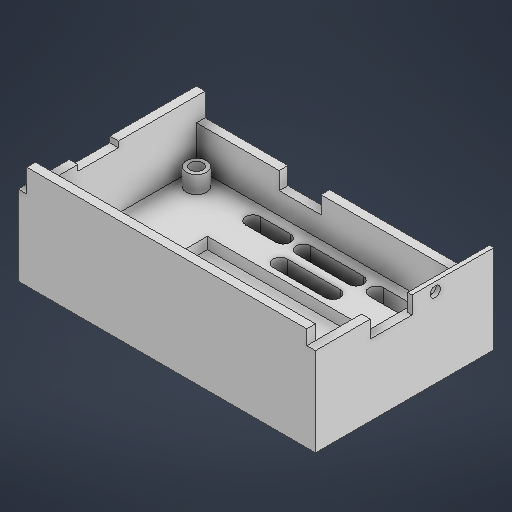
# Autodesk Inventor part: krabice
Saved by Autodesk Inventor 2025 (Build 290162000, 162)
## iProperties
Created: 2025-01-29
Part Number: krabice
Material: Všeobecné
Document SubType Name: Modeling
Designer: psutk
Density: 1 g/cm^3
Appearance: Výchozí
Author: psutk
Autodesk Inventor part; units mm, degrees
ref_plane "YZ Plane" through (0, 0, 0) normal (1, 0, 0) x (0, 1, 0)
ref_plane "XZ Plane" through (0, 0, 0) normal (0, 1, 0) x (-1, 0, 0)
ref_plane "XY Plane" through (0, 0, 0) normal (0, 0, 1) x (1, 0, 0)
sketch "Náčrt1" plane through (0, 0, 0) normal (0, 0, 1) x (1, 0, 0)
  line L0 (-47.25, 26.75) -> (47.25, 26.75)
  line L1 (47.25, 26.75) -> (47.25, -26.75)
  line L2 (47.25, -26.75) -> (-47.25, -26.75)
  line L3 (-47.25, -26.75) -> (-47.25, 26.75)
  line L4 (0, 43.05) -> (0, -43.05) projected
  line L5 (-71.75, 0) -> (71.75, 0) projected
  line L6 (51.25, 30.75) -> (-51.25, 30.75)
  line L7 (-51.25, 30.75) -> (-51.25, -30.75)
  line L8 (-51.25, -30.75) -> (51.25, -30.75)
  line L9 (51.25, -30.75) -> (51.25, 30.75)
  point P0 (0, 0)
  dimension "d0" = 94.5
  dimension "d1" = 53.5
  dimension "d2" = 4
  constraints: 16 end point, 4 parallel, 2 perpendicular, 1 horizontal, 5 other
  measures "d0" distance of L1.end L2.end
  measures "d1" distance of L0.end L1.end
  measures "d2" distance between parallel lines of L0 L6
extrude "Vysunutí1" add sketch "Náčrt1" along normal blind 4
sketch "Náčrt5" plane through (0, 0, 0) normal (0, 0, -1) x (-1, 0, 0)
  line L0 (51.25, -30.75) -> (-51.25, -30.75) projected
  line L1 (-51.25, -30.75) -> (-51.25, 30.75) projected
  line L2 (51.25, -30.75) -> (-51.25, -30.75)
  line L3 (-51.25, -30.75) -> (-51.25, 30.75)
  line L4 (-51.25, 30.75) -> (51.25, 30.75)
  line L5 (51.25, 30.75) -> (51.25, -30.75)
  line L6 (51.25, -30.75) -> (-51.25, -30.75) projected
  line L7 (51.25, 30.75) -> (51.25, -30.75) projected
  line L8 (-51.25, 30.75) -> (51.25, 30.75) projected
  line L9 (-51.25, -30.75) -> (-51.25, 30.75) projected
  point P0 (0, 0)
  point P1 (42.75, -22.25)
  constraints: 8 end point, 2 parallel, 1 horizontal, 1 perpendicular
extrude "Vysunutí4" add sketch "Náčrt5" along normal blind 2
sketch "Náčrt7" plane through (0, 0, 4) normal (0, 0, 1) x (1, 0, 0)
  line L0 (-51.25, -30.75) -> (51.25, -30.75) projected
  line L1 (51.25, -30.75) -> (51.25, 30.75) projected
  line L2 (51.25, 30.75) -> (-51.25, 30.75) projected
  line L3 (-51.25, 30.75) -> (-51.25, -30.75) projected
  line L4 (-48.25, 27.75) -> (48.25, 27.75)
  line L5 (48.25, 27.75) -> (48.25, -27.75)
  line L6 (48.25, -27.75) -> (-48.25, -27.75)
  line L7 (-48.25, -27.75) -> (-48.25, 27.75)
  point P0 (0, 0)
  dimension "d44" = 61.5
  dimension "d45" = 102.5
  dimension "d46" = 3
  dimension "d47" = 3
  dimension "d48" = 3
  dimension "d49" = 3
  constraints: 8 end point, 2 parallel, 1 horizontal, 1 perpendicular
  measures "d44" distance of L2.end L0.start
  measures "d45" distance of L1.end L2.end
  measures "d46" distance between parallel lines of L2 L4
  measures "d47" distance between parallel lines of L3 L7
  measures "d48" distance between parallel lines of L1 L5
  measures "d49" distance between parallel lines of L0 L6
extrude "Vysunutí5" add sketch "Náčrt7" along normal blind 7.5
sketch "Náčrt8" plane through (0, 0, 11.5) normal (0, 0, 1) x (1, 0, 0)
  line L0 (48.25, -27.75) -> (48.25, 27.75) projected
  line L1 (-51.25, 30.75) -> (51.25, 30.75) projected
  line L2 (48.25, 27.75) -> (-5.34, 27.75)
  line L3 (-5.34, 27.75) -> (-5.34, 30.75)
  line L4 (-5.34, 30.75) -> (48.25, 30.75)
  line L5 (48.25, 30.75) -> (48.25, 27.75)
  line L6 (48.25, 27.75) -> (-48.25, 27.75) projected
  line L7 (-48.25, 27.75) -> (-19.76, 27.75)
  line L8 (-19.76, 27.75) -> (-19.76, 30.75)
  line L9 (-19.76, 30.75) -> (-48.25, 30.75)
  line L10 (-48.25, 30.75) -> (-48.25, 27.75)
  point P0 (0, 0)
  dimension "d52" = 53.59
  dimension "d53" = 28.49
  constraints: 16 end point, 4 parallel, 2 horizontal, 2 perpendicular, 2 point on line
  measures "d52" distance of L3.end L4.end
  measures "d53" distance of L9.end L8.end
extrude "Vysunutí6" add sketch "Náčrt8" along normal blind 6 contours L1 L8 L6 L10 | L1 L5 L2 L3
sketch "Náčrt9" plane through (0, 0, 11.5) normal (0, 0, 1) x (1, 0, 0)
  line L0 (51.25, -30.75) -> (51.25, 30.75) projected
  line L1 (51.25, 30.75) -> (48.25, 30.75) projected
  line L2 (51.25, -30.75) -> (48.25, -30.75)
  line L3 (48.25, -30.75) -> (48.25, 30.75)
  line L4 (48.25, 30.75) -> (51.25, 30.75)
  line L5 (51.25, 30.75) -> (51.25, -30.75)
  point P0 (0, 0)
  constraints: 8 end point, 2 parallel, 1 horizontal, 1 perpendicular
extrude "Vysunutí7" add sketch "Náčrt9" along normal blind 11
sketch "Náčrt10" plane through (0, 0, 22.5) normal (0, 0, 1) x (1, 0, 0)
  line L0 (48.25, 30.75) -> (48.25, -30.75) projected
  line L1 (51.25, -30.75) -> (51.25, 30.75) projected
  line L2 (48.25, -11.888) -> (51.25, -11.888)
  line L3 (51.25, -11.888) -> (51.25, 2.532)
  line L4 (51.25, 2.532) -> (48.25, 2.532)
  line L5 (48.25, 2.532) -> (48.25, -11.888)
  line L6 (48.25, -4.678) -> (51.25, -4.678)
  line L7 (48.25, -30.75) -> (51.25, -30.75)
  line L8 (51.25, -30.75) -> (51.25, -11.888)
  line L9 (51.25, -11.888) -> (48.25, -11.888)
  line L10 (48.25, -11.888) -> (48.25, -30.75)
  line L11 (48.25, 2.532) -> (51.25, 2.532)
  line L12 (51.25, 2.532) -> (51.25, 30.75)
  line L13 (51.25, 30.75) -> (48.25, 30.75)
  line L14 (48.25, 30.75) -> (48.25, 2.532)
  point P0 (0, 0)
  dimension "d58" = 26.072
  dimension "d59" = 14.42
  constraints: 26 end point, 6 parallel, 4 perpendicular, 3 horizontal, 3 point on line, 1 midpoint, 1 other
  measures "d58" distance of L0.end L6.start
  measures "d59" distance of L3.end L2.end
extrude "Vysunutí8" add sketch "Náčrt10" along normal blind 6 contours L13 L1 L4 L0 | L2 L1 L7 L0
sketch "Náčrt11" plane through (0, 0, 11.5) normal (0, 0, 1) x (1, 0, 0)
  line L0 (-51.25, -30.75) -> (48.25, -30.75) projected
  line L1 (-48.25, 30.75) -> (-48.25, 27.75) projected
  line L2 (-51.25, -30.75) -> (-48.25, -30.75)
  line L3 (-48.25, -30.75) -> (-48.25, 30.75)
  line L4 (-48.25, 30.75) -> (-51.25, 30.75)
  line L5 (-51.25, 30.75) -> (-51.25, -30.75)
  point P0 (0, 0)
  constraints: 8 end point, 2 parallel, 1 horizontal, 1 perpendicular
extrude "Vysunutí9" add sketch "Náčrt11" along normal blind 12
sketch "Náčrt12" plane through (0, 0, 23.5) normal (0, 0, 1) x (1, 0, 0)
  line L0 (-51.25, -30.75) -> (-48.25, -30.75) projected
  line L1 (-48.25, -30.75) -> (-48.25, 30.75) projected
  line L2 (-48.25, 30.75) -> (-51.25, 30.75) projected
  line L3 (-51.25, 30.75) -> (-51.25, -30.75) projected
  line L4 (-48.25, -6.14) -> (-51.25, -6.14)
  line L5 (-48.25, 0.86) -> (-51.25, 0.86)
  line L6 (-51.25, 0.86) -> (-51.25, -13.14)
  line L7 (-51.25, -13.14) -> (-48.25, -13.14)
  line L8 (-48.25, -13.14) -> (-48.25, 0.86)
  line L9 (-48.25, 30.75) -> (-51.25, 30.75)
  line L10 (-51.25, 30.75) -> (-51.25, 0.86)
  line L11 (-51.25, 0.86) -> (-48.25, 0.86)
  line L12 (-48.25, 0.86) -> (-48.25, 30.75)
  line L13 (-48.25, -13.14) -> (-51.25, -13.14)
  line L14 (-51.25, -13.14) -> (-51.25, -30.75)
  line L15 (-51.25, -30.75) -> (-48.25, -30.75)
  line L16 (-48.25, -30.75) -> (-48.25, -13.14)
  point P0 (0, 0)
  point P1 (-48.25, -13.14)
  point P2 (-51.25, 0.86)
  dimension "d64" = 24.61
  dimension "d65" = 14
  constraints: 26 end point, 6 parallel, 4 perpendicular, 4 point on line, 3 horizontal, 1 other
  measures "d64" distance from line of L0 L4.start
  measures "d65" distance of L6.end L5.end
extrude "Vysunutí10" add sketch "Náčrt12" along normal blind 2 contours L3 L7 L1 L0 | L3 L2 L1 L5
sketch "Náčrt13" plane through (0, 0, 11.5) normal (0, 0, 1) x (1, 0, 0)
  line L0 (-48.25, -30.75) -> (48.25, -30.75) projected
  line L1 (-48.25, -30.75) -> (48.25, -30.75)
  line L2 (48.25, -30.75) -> (48.25, -27.75)
  line L3 (48.25, -27.75) -> (-48.25, -27.75)
  line L4 (-48.25, -27.75) -> (-48.25, -30.75)
  point P0 (0, 0)
  constraints: 8 end point, 2 parallel, 1 horizontal, 1 perpendicular
extrude "Vysunutí11" add sketch "Náčrt13" along normal blind 17
sketch "Náčrt14" plane through (0, 0, 4) normal (0, 0, 1) x (1, 0, 0)
  line L0 (-48.25, 27.75) -> (-48.25, -27.75) projected
  line L1 (-48.25, -27.75) -> (48.25, -27.75) projected
  line L2 (48.25, -27.75) -> (48.25, 27.75) projected
  line L3 (48.25, 27.75) -> (-48.25, 27.75) projected
  line L4 (0, 43.05) -> (0, -43.05) projected
  line L5 (-71.75, 0) -> (71.75, 0) projected
  line L6 (39.75, -20.5179) -> (42.75, -18.7859)
  line L7 (42.75, -18.7859) -> (45.75, -20.5179)
  line L8 (45.75, -20.5179) -> (45.75, -23.9821)
  line L9 (45.75, -23.9821) -> (42.75, -25.7141)
  line L10 (42.75, -25.7141) -> (39.75, -23.9821)
  line L11 (39.75, -23.9821) -> (39.75, -20.5179)
  point P0 (0, 0)
  point P1 (42.75, -22.25)
  point P2 (-42.75, -22.25)
  point P3 (-42.75, 22.25)
  point P4 (42.75, 22.25)
  point P5 (42.75, -22.25)
  dimension "d70" = 5.5
  dimension "d71" = 5.5
  dimension "d72" = 6
  constraints: 12 end point, 3 symmetric about line, 1 coincident, 13 other
  measures "d70" distance from line of L1 point (42.75, -22.25)
  measures "d71" distance from line of L2 point (42.75, -22.25)
  measures "d72" distance between parallel lines of L8 L11
extrude "Vysunutí12" cut sketch "Náčrt14" along normal blind 4 from surface at -6 contours L6 L7 L8 L9 L10 L11
pattern_linear "Obdélníkové pole3" count 2 spacing 85.5 along (-1, 0, 0) count 2 spacing 44.5 along (0, 1, 0) of "Vysunutí12"
sketch "Náčrt16" plane through (0, 0, 4) normal (0, 0, 1) x (1, 0, 0)
  circle A0 centre (42.75, -22.25) radius 1.7 projected
  circle A1 centre (42.75, -22.25) radius 3.5
  point P0 (0, 0)
  dimension "d115" = 7
  constraints: 2 coincident, 1 centre point
  measures "d115" diameter of A1
extrude "Vysunutí13" add sketch "Náčrt16" along normal blind 6 contours A0 | A1
pattern_linear "Obdélníkové pole5" count 2 spacing 85.5 along (-1, 0, 0) count 2 spacing 44.5 along (0, 1, 0) of "Vysunutí13"
sketch "Náčrt17" plane through (0, 0, 10) normal (0, 0, 1) x (1, 0, 0)
  line L0 (39.5, -24.1264) -> (42.75, -26.0028) projected
  line L1 (42.75, -26.0028) -> (46, -24.1264) projected
  line L2 (46, -24.1264) -> (46, -20.3736) projected
  line L3 (46, -20.3736) -> (42.75, -18.4972) projected
  line L4 (42.75, -18.4972) -> (39.5, -20.3736) projected
  line L5 (39.5, -20.3736) -> (39.5, -24.1264) projected
  point P0 (0, 0)
  point P1 (42.75, -22.25)
hole "Díra4" at (42.75, -22.25, 10) direction (0, 0, -1) diameter 4.4 end through all
pattern_linear "Obdélníkové pole6" count 2 spacing 85.5 along (-1, 0, 0) count 2 spacing 44.5 along (0, 1, 0) of "Díra4"
sketch "Náčrt18" plane through (0, 0, 28.5) normal (0, 0, 1) x (1, 0, 0)
  line L0 (51.25, -30.75) -> (51.25, -11.888) projected
  line L1 (51.25, -11.888) -> (48.25, -11.888) projected
  line L2 (48.25, -11.888) -> (48.25, -27.75) projected
  line L3 (48.25, -27.75) -> (-48.25, -27.75) projected
  line L4 (-48.25, -27.75) -> (-48.25, -30.75) projected
  line L5 (-48.25, -30.75) -> (51.25, -30.75) projected
  line L6 (48.25, -27.75) -> (-48.25, -27.75)
  line L7 (-48.25, -27.75) -> (-48.25, -30.75)
  line L8 (-48.25, -30.75) -> (48.25, -30.75)
  line L9 (48.25, -30.75) -> (48.25, -27.75)
  point P0 (0, 0)
  constraints: 8 end point, 2 parallel, 1 horizontal, 1 perpendicular
extrude "Vysunutí14" add sketch "Náčrt18" along normal blind 5 contours L5 L4 L3 L9
sketch "Náčrt19" plane through (48.25, -27.75, 4) normal (-1, 0, 0) x (0, 0, 1)
  line L0 (24.5, 58.5) -> (24.5, 30.282) projected
  line L1 (24.5, 30.282) -> (18.5, 30.282)
  line L2 (18.5, 30.282) -> (18.5, 58.5)
  line L3 (18.5, 58.5) -> (24.5, 58.5)
  line L4 (24.5, 58.5) -> (24.5, 30.282)
  point P0 (-4, 27.75)
  dimension "d118" = 6
  dimension "d130" = 28.218
  constraints: 8 end point, 2 parallel, 1 horizontal, 1 perpendicular
  measures "d118" distance of L2.end L3.end
  measures "d130" distance of L1.end L2.end
extrude "Vysunutí15" cut sketch "Náčrt19" against normal blind 1.5
sketch "Náčrt20" plane through (51.25, -30.75, -2) normal (1, 0, 0) x (0, 0, -1)
  line L0 (-24.5, 33.282) -> (-24.5, 61.5) projected
  line L1 (0, 61.5) -> (-30.5, 61.5) projected
  line L2 (-30.5, 33.282) -> (-30.5, 61.5) projected
  line L3 (-24.5, 33.282) -> (-30.5, 33.282) projected
  line L4 (-24.5, 18.862) -> (-24.5, 33.282) projected
  line L5 (-24.5, 18.862) -> (-30.5, 18.862) projected
  line L6 (-30.5, 0) -> (-30.5, 18.862) projected
  line L7 (0, 0) -> (-30.5, 0) projected
  line L8 (0, 61.5) -> (0, 0) projected
  point P0 (-2, 30.75)
  point P1 (-24.5, 58.5)
  point P2 (-27.5, 41.282)
  dimension "d121" = 3
  dimension "d122" = 8
  measures "d121" distance from line of L2 point (-27.5, 41.282)
  measures "d122" distance from line of L3 point (-27.5, 41.282)
hole "Díra5" at (51.25, 10.532, 25.5) direction (-1, 0, 0) diameter 3.6 depth 1.5 clearance for "Šroub se zápustnou hlavou ISO 2009/7046" size "M3" standard "ISO"
sketch "Náčrt21" plane through (0, 0, 4) normal (0, 0, 1) x (1, 0, 0)
  line L0 (35.25, 21.75) -> (19.71, 21.75) construction
  line L1 (35.25, 24.25) -> (19.71, 24.25)
  line L2 (19.71, 19.25) -> (35.25, 19.25)
  arc A0 (35.25, 19.25) -> (35.25, 24.25) centre (35.25, 21.75) ccw
  arc A1 (19.71, 24.25) -> (19.71, 19.25) centre (19.71, 21.75) ccw
  line L3 (-5.34, 27.75) -> (48.25, 27.75) projected
  line L4 (48.25, 30.75) -> (48.25, -11.888) projected
  point P0 (0, 0)
  point P1 (27.48, 21.75)
  point P2 (37.75, 21.75)
  point P3 (17.21, 21.75)
  dimension "d132" = 5
  dimension "d133" = 6
  dimension "d134" = 13
  dimension "d154" = 20.54
  constraints: 8 end point, 6 point on circle, 4 tangent, 2 centre point, 1 horizontal, 1 midpoint, 1 parallel
  measures "d132" diameter of A1
  measures "d133" distance between parallel lines of L3 L0
  measures "d134" distance from line of L4 L0.start
  measures "d154" distance of point (37.75, 21.75) point (17.21, 21.75)
extrude "Vysunutí16" cut sketch "Náčrt21" against normal blind 10
sketch "Náčrt22" plane through (0, 0, 4) normal (0, 0, 1) x (1, 0, 0)
  line L0 (12.71, 21.75) -> (-5.37, 21.75) construction
  line L1 (12.71, 24.25) -> (-5.37, 24.25)
  line L2 (-5.37, 19.25) -> (12.71, 19.25)
  arc A0 (12.71, 19.25) -> (12.71, 24.25) centre (12.71, 21.75) ccw
  arc A1 (-5.37, 24.25) -> (-5.37, 19.25) centre (-5.37, 21.75) ccw
  line L3 (35.25, 19.25) -> (19.71, 19.25) projected
  arc A2 (19.71, 24.25) -> (19.71, 19.25) centre (19.71, 21.75) ccw projected
  line L4 (-5.34, 27.75) -> (48.25, 27.75) projected
  point P0 (0, 0)
  point P1 (3.67, 21.75)
  point P2 (17.21, 21.75)
  point P3 (15.21, 21.75)
  point P4 (-7.87, 21.75)
  dimension "d137" = 5
  dimension "d139" = 2
  dimension "d155" = 3.5
  dimension "d156" = 23.08
  constraints: 8 end point, 7 point on circle, 4 tangent, 2 centre point, 1 horizontal, 1 midpoint, 1 parallel
  measures "d137" diameter of A1
  measures "d139" distance of point (17.21, 21.75) point (15.21, 21.75)
  measures "d155" distance between parallel lines of L4 L1
  measures "d156" distance of point (15.21, 21.75) point (-7.87, 21.75)
extrude "Vysunutí17" cut sketch "Náčrt22" against normal blind 10
pattern_linear "Obdélníkové pole7" count 2 spacing 8 along (0, -1, 0) of "Vysunutí17"
sketch "Náčrt23" plane through (0, 0, 4) normal (0, 0, 1) x (1, 0, 0)
  line L0 (-12.37, 21.75) -> (-22.83, 21.75) construction
  line L1 (-12.37, 24.25) -> (-22.83, 24.25)
  line L2 (-22.83, 19.25) -> (-12.37, 19.25)
  arc A0 (-12.37, 19.25) -> (-12.37, 24.25) centre (-12.37, 21.75) ccw
  arc A1 (-22.83, 24.25) -> (-22.83, 19.25) centre (-22.83, 21.75) ccw
  arc A2 (-5.37, 24.25) -> (-5.37, 19.25) centre (-5.37, 21.75) ccw projected
  circle A3 centre (-42.75, 22.25) radius 3.5 projected
  line L3 (-48.25, 27.75) -> (-19.76, 27.75) projected
  point P0 (0, 0)
  point P1 (-17.6, 21.75)
  point P2 (-7.87, 21.75)
  point P3 (-9.87, 21.75)
  point P4 (-25.33, 21.75)
  point P5 (-7.87, 21.75)
  dimension "d146" = 5
  dimension "d150" = 2
  dimension "d151" = 3.5
  dimension "d157" = 15.46
  constraints: 8 end point, 8 point on circle, 4 tangent, 2 centre point, 1 horizontal, 1 midpoint, 1 parallel
  measures "d146" diameter of A1
  measures "d150" distance of point (-7.87, 21.75) point (-9.87, 21.75)
  measures "d151" distance between parallel lines of L3 L1
  measures "d157" distance of point (-9.87, 21.75) point (-25.33, 21.75)
extrude "Vysunutí18" cut sketch "Náčrt23" against normal blind 10 contours A0 L2 A1 L1
sketch "Náčrt24" plane through (0, 0, -2) normal (0, 0, -1) x (-1, 0, 0)
  line L0 (-26, 9.25) -> (26, 9.25)
  line L1 (26, 9.25) -> (26, -27.75)
  line L2 (26, -27.75) -> (-26, -27.75)
  line L3 (-26, -27.75) -> (-26, 9.25)
  line L4 (0, -43.05) -> (0, 43.05) projected
  line L5 (-71.75, 0) -> (71.75, 0) projected
  line L6 (48.25, -27.75) -> (-48.25, -27.75) projected
  point P0 (0, 0)
  dimension "d159" = 52
  dimension "d164" = 37
  constraints: 8 end point, 2 parallel, 1 collinear, 1 horizontal, 1 perpendicular, 1 other
  measures "d159" distance of L1.end L2.end
  measures "d164" distance between parallel lines of L2 L0
extrude "Vysunutí19" cut sketch "Náčrt24" along normal blind 4 from surface at -6
